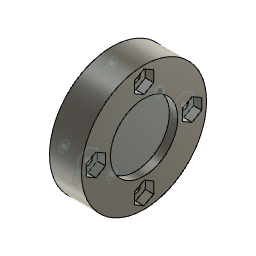
Coupling_1 v1 (Autodesk Fusion 360 design; units mm, degrees)
Autodesk Fusion 360 part; units mm, degrees
sketch "Sketch1" plane through (0, 0, 0) normal (1, 0, 0) x (0, 1, 0)
  circle A0 centre (0, 0) radius 19.5
  dimension "d1" = 39
  constraint coincident A0.centre origin
  measures "d1" diameter of A0
extrude "Extrude1" add sketch "Sketch1" along normal blind 10
sketch "Sketch2" plane through (0, 0, 0) normal (1, 0, 0) x (0, 1, 0)
  line L0 (5.8998, 1.1158) -> (1.9836, 5.6673)
  line L1 (1.9836, 5.6673) -> (-3.9163, 4.5515)
  line L2 (-3.9163, 4.5515) -> (-5.8998, -1.1158)
  line L3 (-5.8998, -1.1158) -> (-1.9836, -5.6673)
  line L4 (-1.9836, -5.6673) -> (3.9163, -4.5515)
  line L5 (3.9163, -4.5515) -> (5.8998, 1.1158)
  dimension "d4" = 5.2
  measures "d4" distance of origin L5
extrude "Extrude2" cut sketch "Sketch2" along normal blind 4.2
sketch "Sketch3" plane through (10, 0, 0) normal (1, 0, 0) x (0, 1, 0)
  circle A0 centre (0, 0) radius 19.5
  circle A1 centre (0, 0) radius 10.5
  dimension "d7" = 21
  constraint concentric A0 A1
  measures "d7" diameter of A1
extrude "Extrude3" cut sketch "Sketch3" against normal blind 2.6 contours A1
sketch "Sketch4" plane through (0, 0, 0) normal (1, 0, 0) x (0, 1, 0)
sketch "Sketch5" plane through (0, 0, 0) normal (1, 0, 0) x (0, 1, 0)
  circle A0 centre (0, -15) radius 1.5
  dimension "d10" = 3
  measures "d10" diameter of A0
sketch "Sketch6" plane through (0, 0, 0) normal (1, 0, 0) x (0, 1, 0)
  circle A0 centre (-14, 0) radius 1.5
  circle A1 centre (0, 14) radius 1.5
  circle A2 centre (14, 0) radius 1.5
  dimension "d13" = 3
  dimension "d14" = 3
  dimension "d15" = 3
  measures "d13" diameter of A0
  measures "d14" diameter of A1
  measures "d15" diameter of A2
sketch "Sketch7" plane through (0, 0, 0) normal (-1, 0, 0) x (0, -1, 0)
  line L0 (1.9836, -5.6673) -> (-3.9163, -4.5515)
  line L1 (-3.9163, -4.5515) -> (-5.8998, 1.1158)
  line L2 (-5.8998, 1.1158) -> (-1.9836, 5.6673)
  line L3 (-1.9836, 5.6673) -> (3.9163, 4.5515)
  line L4 (3.9163, 4.5515) -> (5.8998, -1.1158)
  line L5 (5.8998, -1.1158) -> (1.9836, -5.6673)
  circle A0 centre (0, 0) radius 19.5
  circle A1 centre (0, 15) radius 1.5
  circle A2 centre (-15, 0) radius 1.5
  point P0 (-15, 0)
  dimension "d18" = 3
  dimension "d28" = 3
  constraint coincident P0 A2.centre
  measures "d18" diameter of A1
  measures "d28" diameter of A2
sketch "Sketch8" plane through (0, 0, 0) normal (1, 0, 0) x (0, 1, 0)
  circle A0 centre (-15, 0) radius 1.5
  dimension "d21" = 3
  measures "d21" diameter of A0
extrude "Extrude7" cut sketch "Sketch8" along normal blind 12
extrude "Extrude8" cut sketch "Sketch5" along normal blind 15
extrude "Extrude9" cut sketch "Sketch7" against normal blind 15 contours A1
extrude "Extrude10" cut sketch "Sketch7" against normal blind 15 contours A2
sketch "Sketch10" plane through (7.4, 0, 0) normal (1, 0, 0) x (0, 1, 0)
  circle A0 centre (0, 0) radius 10.5
  line L0 (-3.003, -16.7268) -> (-0.0431, -18.5265)
  line L1 (-0.0431, -18.5265) -> (2.9955, -16.8631)
  line L2 (2.9955, -16.8631) -> (3.0742, -13.3999)
  line L3 (3.0742, -13.3999) -> (0.1143, -11.6001)
  line L4 (0.1143, -11.6001) -> (-2.9243, -13.2636)
  line L5 (-2.9243, -13.2636) -> (-3.003, -16.7268)
  point P0 (0.0356, -15.0633)
  dimension "d32" = 3
  measures "d32" distance of P0 L5
extrude "Extrude11" cut sketch "Sketch10" along normal blind 2600 contours L0 L1 L2 L3 L4 L5
sketch "Sketch11" plane through (7.4, 0, 0) normal (1, 0, 0) x (0, 1, 0)
  circle A0 centre (0, 0) radius 10.5
  line L0 (-18, -1.7321) -> (-15, -3.4641)
  line L1 (-15, -3.4641) -> (-12, -1.7321)
  line L2 (-12, -1.7321) -> (-12, 1.7321)
  line L3 (-12, 1.7321) -> (-15, 3.4641)
  line L4 (-15, 3.4641) -> (-18, 1.7321)
  line L5 (-18, 1.7321) -> (-18, -1.7321)
  point P0 (-15, 0)
  dimension "d35" = 3
  measures "d35" distance of P0 L5
extrude "Extrude12" cut sketch "Sketch11" along normal blind 2.6 contours L0 L1 L2 L3 L4 L5
sketch "Sketch13" plane through (7.4, 0, 0) normal (1, 0, 0) x (0, 1, 0)
  circle A0 centre (0, 0) radius 10.5
  line L0 (3, 16.7321) -> (0, 18.4641)
  line L1 (0, 18.4641) -> (-3, 16.7321)
  line L2 (-3, 16.7321) -> (-3, 13.2679)
  line L3 (-3, 13.2679) -> (0, 11.5359)
  line L4 (0, 11.5359) -> (3, 13.2679)
  line L5 (3, 13.2679) -> (3, 16.7321)
  point P0 (0, 15)
  dimension "d39" = 3
  measures "d39" distance of P0 L5
extrude "Extrude13" cut sketch "Sketch13" along normal blind 2.6 contours L0 L1 L2 L3 L4 L5
sketch "Sketch14" plane through (7.4, 0, 0) normal (1, 0, 0) x (0, 1, 0)
  circle A0 centre (0, 0) radius 10.5
  line L0 (12, -1.7321) -> (15, -3.4641)
  line L1 (15, -3.4641) -> (18, -1.7321)
  line L2 (18, -1.7321) -> (18, 1.7321)
  line L3 (18, 1.7321) -> (15, 3.4641)
  line L4 (15, 3.4641) -> (12, 1.7321)
  line L5 (12, 1.7321) -> (12, -1.7321)
  point P0 (15, 0)
extrude "Extrude14" cut sketch "Sketch14" along normal blind 2.6 contours L0 L1 L2 L3 L4 L5
sketch "Sketch15" plane through (7.4, 0, 0) normal (1, 0, 0) x (0, 1, 0)
